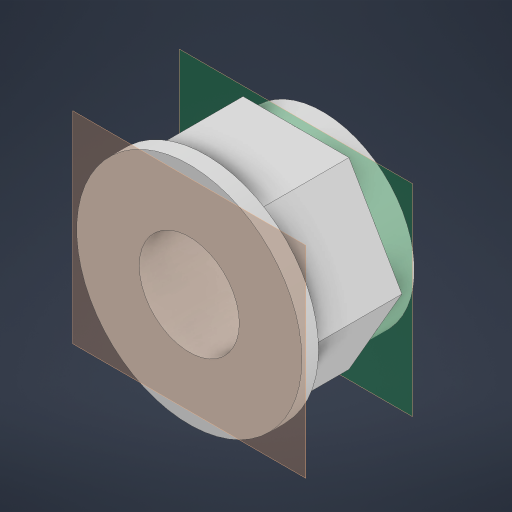
# Autodesk Inventor part: locknut
Saved by Autodesk Inventor 2023 (Build 270158000, 158)
## iProperties
Created: 2023-12-15
Part Number: locknut
Material: 一般
Document SubType Name: Modeling
Designer: IshiiLabHonda
Density: 1 g/cm^3
Appearance: 既定
Author: IshiiLabHonda
Autodesk Inventor part; units mm, degrees
ref_plane "YZ Plane" through (0, 0, 0) normal (1, 0, 0) x (0, 1, 0)
ref_plane "XZ Plane" through (0, 0, 0) normal (0, 1, 0) x (-1, 0, 0)
ref_plane "XY Plane" through (0, 0, 0) normal (0, 0, 1) x (1, 0, 0)
sketch "スケッチ1" plane through (0, 0, 0) normal (0, 0, 1) x (1, 0, 0)
  line L0 (3.1754, 0) -> (1.5877, -2.75)
  line L1 (1.5877, -2.75) -> (-1.5877, -2.75)
  line L2 (-1.5877, -2.75) -> (-3.1754, 0)
  line L3 (-3.1754, 0) -> (-1.5877, 2.75)
  line L4 (-1.5877, 2.75) -> (1.5877, 2.75)
  line L5 (1.5877, 2.75) -> (3.1754, 0)
  point P0 (0, 0)
  point P1 (0, 0)
  dimension "d0" = 5.5
  constraints: 12 end point, 1 coincident, 13 other
  measures "d0" distance between parallel lines of L0 L3
extrude "押し出し1" add sketch "スケッチ1" along normal blind 3.2
ref_plane "作業平面1" through (0, 0, 0) normal (0, 0, -1) x (-1, 0, 0)
sketch "スケッチ3" plane through (0, 0, 0) normal (0, 0, -1) x (-1, 0, 0)
  circle A0 centre (0, 0) radius 2.75
  line L0 (3.1754, 0) -> (1.5877, -2.75) projected
  constraints: 1 centre point, 1 coincident, 1 tangent
extrude "押し出し3" add sketch "スケッチ3" along normal blind 0.8
sketch "スケッチ2" plane through (0, 0, 0) normal (0, 0, 1) x (1, 0, 0)
  circle A0 centre (0, 0) radius 1.5
  dimension "d3" = 3
  constraints: 1 centre point, 1 coincident
  measures "d3" diameter of A0
extrude "押し出し2" cut sketch "スケッチ2" along normal mid plane 10
ref_plane "作業平面2" through (0, 0, 3.2) normal (0, 0, 1) x (1, 0, 0)
sketch "スケッチ4" plane through (0, 0, 3.2) normal (0, 0, 1) x (1, 0, 0)
  circle A0 centre (0, 0) radius 3.3754
  circle A1 centre (0, 0) radius 1.5 projected
  line L0 (1.5877, 2.75) -> (-1.5877, 2.75) projected
  line L1 (-1.5877, 2.75) -> (-3.1754, 0) projected
  line L2 (-3.1754, 0) -> (-1.5877, -2.75) projected
  line L3 (-1.5877, -2.75) -> (1.5877, -2.75) projected
  line L4 (1.5877, -2.75) -> (3.1754, 0) projected
  line L5 (3.1754, 0) -> (1.5877, 2.75) projected
  circle A2 centre (0, 0) radius 3.1754
  dimension "d10" = 0.2
  constraints: 2 coincident, 1 centre point, 3 other
extrude "押し出し4" add sketch "スケッチ4" against normal blind 0.5 contours A0 | A2 L5 | L0 A2 | L1 A2 | A2 L4 | L2 A2 | A2 L3
